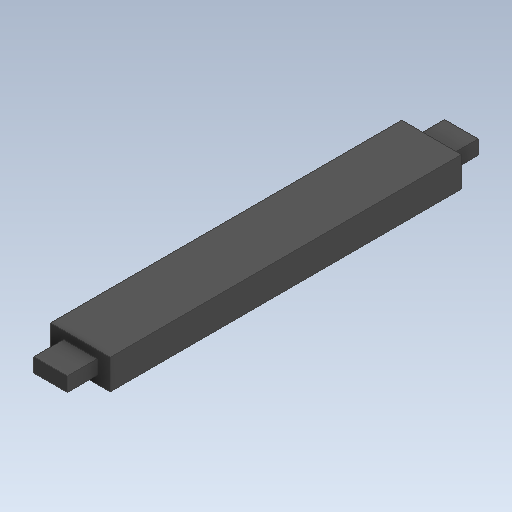
# Autodesk Inventor part: spool holder span
Saved by Autodesk Inventor 2020.2 (Build 242310000, 310)
## iProperties
Created: 2020-02-09
Part Number: spool holder span
Material: PLA
Document SubType Name: Modeling
Designer: mulve
Density: 1.3 g/cm^3
Appearance: Generic
Mass: 33.5776 g
Surface Area: 83.6924 cm^2
Volume: 25.829 cm^3
Author: mulve
Autodesk Inventor part; units mm, degrees
ref_plane "YZ Plane" through (0, 0, 0) normal (1, 0, 0) x (0, 1, 0)
ref_plane "XZ Plane" through (0, 0, 0) normal (0, 1, 0) x (-1, 0, 0)
ref_plane "XY Plane" through (0, 0, 0) normal (0, 0, 1) x (1, 0, 0)
sketch "Sketch1" plane through (0, 0, 0) normal (0, 1, 0) x (-1, 0, 0)
  line L0 (0, 0) -> (20.32, 0)
  line L1 (20.32, 0) -> (20.32, -140)
  line L2 (20.32, -140) -> (0, -140)
  line L3 (0, -140) -> (0, 0)
  dimension "d0" = 140
  dimension "d1" = 20.32
  constraints: 8 end point, 2 parallel, 1 horizontal, 1 perpendicular
  measures "d0" distance of L0.end L1.end
  measures "d1" distance of L1.end L2.end
extrude "Extrusion1" add sketch "Sketch1" along normal blind 10.16
sketch "Sketch2" plane through (-20.32, 0, 0) normal (0, 0, 1) x (1, 0, 0)
  line L0 (4.445, 7.493) -> (15.875, 7.493)
  line L1 (15.875, 7.493) -> (15.875, 2.667)
  line L2 (15.875, 2.667) -> (4.445, 2.667)
  line L3 (4.445, 2.667) -> (4.445, 7.493)
  line L4 (0, 10.16) -> (20.32, 10.16) projected
  line L5 (0, 0) -> (20.32, 0) projected
  line L6 (0, 0) -> (0, 10.16) projected
  line L7 (20.32, 0) -> (20.32, 10.16) projected
  line L8 (0, 10.16) -> (20.32, 10.16)
  line L9 (20.32, 10.16) -> (20.32, 0)
  line L10 (20.32, 0) -> (0, 0)
  line L11 (0, 0) -> (0, 10.16)
  dimension "d4" = 4.826
  dimension "d5" = 11.43
  dimension "d6" = 2.667
  dimension "d7" = 2.667
  dimension "d8" = 4.445
  dimension "d9" = 4.445
  constraints: 16 end point, 4 parallel, 2 horizontal, 2 perpendicular
  measures "d4" distance of L0.end L1.end
  measures "d5" distance of L1.end L2.end
  measures "d6" distance between parallel lines of L4 L0
  measures "d7" distance between parallel lines of L5 L2
  measures "d8" distance between parallel lines of L6 L3
  measures "d9" distance between parallel lines of L7 L1
extrude "Extrusion2" cut sketch "Sketch2" against normal blind 10.16
sketch "Sketch3" plane through (0, 0, -140) normal (0, 0, -1) x (-1, 0, 0)
  line L0 (4.445, 7.493) -> (15.875, 7.493) projected
  line L1 (15.875, 2.667) -> (4.445, 2.667) projected
  line L2 (4.445, 7.493) -> (15.875, 7.493)
  line L3 (15.875, 7.493) -> (15.875, 2.667)
  line L4 (15.875, 2.667) -> (4.445, 2.667)
  line L5 (4.445, 2.667) -> (4.445, 7.493)
  line L6 (20.32, 0) -> (20.32, 10.16) projected
  line L7 (0, 10.16) -> (0, 0) projected
  line L8 (20.32, 10.16) -> (0, 10.16)
  line L9 (0, 10.16) -> (0, 0)
  line L10 (0, 0) -> (20.32, 0)
  line L11 (20.32, 0) -> (20.32, 10.16)
  constraints: 16 end point, 4 parallel, 2 horizontal, 2 perpendicular
extrude "Extrusion3" cut sketch "Sketch3" against normal blind 10.16
equation "\"d6\" = d7"
equation "\"d8\" = d9"
body "Solid1"
